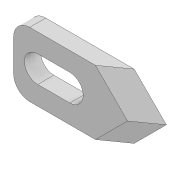
# Autodesk Inventor part: back_lid_mount
Saved by Autodesk Inventor 2022 (Build 260153000, 153)
## iProperties
Created: 2022-05-28
Part Number: back_lid_mount
Material: Generic
Document SubType Name: Modeling
Designer: Thomas
Density: 1 g/cm^3
Appearance: Default
Author: Thomas
Autodesk Inventor part; units mm, degrees
ref_plane "YZ Plane" through (0, 0, 0) normal (1, 0, 0) x (0, 1, 0)
ref_plane "XZ Plane" through (0, 0, 0) normal (0, 1, 0) x (-1, 0, 0)
ref_plane "XY Plane" through (0, 0, 0) normal (0, 0, 1) x (1, 0, 0)
sketch "Sketch1" plane through (0, 0, 0) normal (0, 0, 1) x (1, 0, 0)
  line L0 (0, 0) -> (4, 0) construction
  line L1 (0, -1.65) -> (4, -1.65)
  line L2 (4, 1.65) -> (0, 1.65)
  arc A0 (0, 1.65) -> (0, -1.65) centre (0, 0) ccw
  arc A1 (4, -1.65) -> (4, 1.65) centre (4, 0) ccw
  line L3 (-1, 4) -> (10, 4)
  line L4 (10, -4) -> (-1, -4)
  line L5 (-3, -2) -> (-3, 2)
  arc A2 (-1, 4) -> (-3, 2) centre (-1, 2) ccw
  arc A3 (-3, -2) -> (-1, -4) centre (-1, -2) ccw
  line L6 (10, 4) -> (14, 0)
  line L7 (10, 4) -> (15.6569, 4) construction
  line L8 (14, 0) -> (10, -4)
  point P0 (2, 0)
  point P1 (-3, 4)
  point P2 (-3, -4)
  dimension "d0" = 3.3
  dimension "d1" = 2
  dimension "d2" = 8
  dimension "d3" = 4
  dimension "d4" = 3
  dimension "d5" = 2
  dimension "d6" = 45
  dimension "d7" = 0
  dimension "d8" = 4
  dimension "d9" = 10
  dimension "d10" = 90
  constraints: 20 end point, 8 point on circle, 8 tangent, 4 centre point, 4 point on line, 3 horizontal, 2 parallel, 1 equal length, 1 equal radius, 1 midpoint
  measures "d0" diameter of A1
  measures "d1" distance of point (2, 0) L0.start
  measures "d2" distance of point (-3, -4) point (-3, 4)
  measures "d3" distance from line of L0.start L3
  measures "d4" distance from line of L0.start L5
  measures "d5" radius of A2
  measures "d6" angle of L6 L7
  measures "d7" vertical distance of L6.end L0.start
  measures "d8" distance from line of L0.start L4
  measures "d9" distance of L0.end L6.end
  measures "d10" angle of L6 L8
extrude "Extrusion2" add sketch "Sketch1" along normal blind 2
chamfer "Chamfer1" distance 2 angle 45 2 edges at (12, -2, 2) (12, 2, 2)
equation "\"d3\" = 0.5 * d2"
equation "\"d8\" = d3"
body "Solid2"
